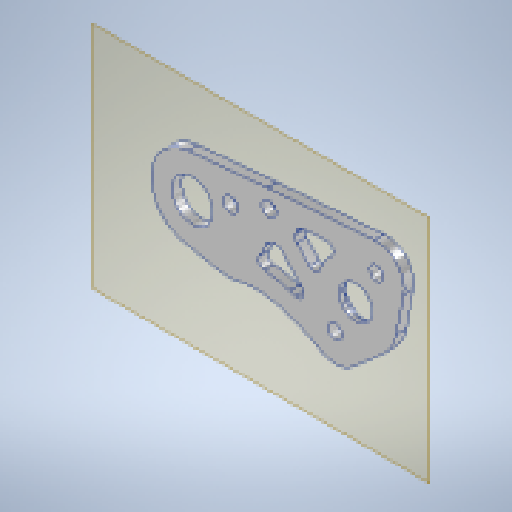
# Autodesk Inventor part: IntakeBearingBlock
Saved by Autodesk Inventor 2023 (Build 270158000, 158)
## iProperties
Created: 2022-11-10
Part Number: IntakeBearingBlock
Material: Aluminum 6061
Document SubType Name: Modeling
Designer: Zac Hah
Density: 2.7 g/cm^3
Appearance: Aluminum - Flat
Author: Zac Hah
Autodesk Inventor part; units mm, degrees
ref_plane "YZ Plane" through (0, 0, 0) normal (1, 0, 0) x (0, 1, 0)
ref_plane "XZ Plane" through (0, 0, 0) normal (0, 1, 0) x (-1, 0, 0)
ref_plane "XY Plane" through (0, 0, 0) normal (0, 0, 1) x (1, 0, 0)
ref_plane "Work Plane1" through (0, 0, 0) normal (0, 0, 1) x (1, 0, 0)
sketch "Sketch1" plane through (0, 0, 0) normal (0, 0, 1) x (1, 0, 0)
  line L0 (44.7498, 2.1658) -> (46.9612, 13.9487) projected
  arc A0 (46.9612, 13.9487) -> (42.8396, 22.8948) centre (38.5982, 15.5182) ccw projected
  arc A1 (42.8396, 22.8948) -> (22.886, 31.7216) centre (-8.8802, -67.0551) ccw projected
  arc A2 (22.886, 31.7216) -> (13.5715, 28.8544) centre (20.2809, 23.6211) ccw projected
  arc A3 (0.8003, 20.1348) -> (13.5715, 28.8544) centre (-6.4566, 44.4761) ccw projected
  line L1 (0.8003, 20.1348) -> (-28.9641, 11.2611) projected
  arc A4 (-28.9641, 11.2611) -> (-47.1072, -13.0801) centre (-21.7072, -13.0801) ccw projected
  line L2 (-47.1072, -13.0801) -> (-47.1072, -25.7801) projected
  arc A5 (-47.1072, -25.7801) -> (-40.7572, -32.1301) centre (-40.7572, -25.7801) ccw projected
  line L3 (-40.7572, -32.1301) -> (-28.0572, -32.1301) projected
  arc A6 (-28.0572, -32.1301) -> (-21.7072, -25.7801) centre (-28.0572, -25.7801) ccw projected
  line L4 (-21.7072, -25.7801) -> (-21.7072, -15.4467) projected
  arc A7 (-19.4393, -12.404) -> (-21.7072, -15.4467) centre (-18.5322, -15.4467) ccw projected
  line L5 (-19.4393, -12.404) -> (-5.7048, -8.3094) projected
  arc A8 (9.7562, -8.6121) -> (-5.7048, -8.3094) centre (1.552, -32.6506) ccw projected
  arc A9 (9.7562, -8.6121) -> (9.8996, -8.6596) centre (12.5046, -0.5592) ccw projected
  arc A10 (21.6959, -13.8779) -> (9.8996, -8.6596) centre (-8.8802, -67.0551) ccw projected
  arc A11 (21.6959, -13.8779) -> (31.501, -12.9394) centre (25.9373, -6.5014) ccw projected
  line L6 (31.501, -12.9394) -> (40.5717, -5.1006) projected
  arc A12 (40.5717, -5.1006) -> (44.7498, 2.1658) centre (32.2678, 4.5084) ccw projected
  arc A13 (29.1025, -0.9965) -> (35.433, 10.0133) centre (32.2678, 4.5084) ccw projected
  arc A14 (29.1025, -0.9965) -> (14.4487, 5.4859) centre (-8.8802, -67.0551) ccw construction
  arc A15 (18.3368, 17.5761) -> (14.4487, 5.4859) centre (16.3928, 11.531) ccw projected
  arc A16 (35.433, 10.0133) -> (18.3368, 17.5761) centre (-8.8802, -67.0551) ccw construction
  arc A17 (24.8611, -8.373) -> (11.8436, -2.6145) centre (-8.8802, -67.0551) ccw construction
  arc A18 (13.1656, 1.4961) -> (11.8436, -2.6145) centre (12.5046, -0.5592) ccw projected
  arc A19 (27.0135, -4.6297) -> (13.1656, 1.4961) centre (-8.8802, -67.0551) ccw construction
  arc A20 (24.8611, -8.373) -> (27.0135, -4.6297) centre (25.9373, -6.5014) ccw projected
  arc A21 (37.5221, 13.6465) -> (39.6744, 17.3899) centre (38.5982, 15.5182) ccw projected
  arc A22 (37.5221, 13.6465) -> (19.6199, 21.5658) centre (-8.8802, -67.0551) ccw construction
  arc A23 (20.9419, 25.6765) -> (19.6199, 21.5658) centre (20.2809, 23.6211) ccw projected
  arc A24 (39.6744, 17.3899) -> (20.9419, 25.6765) centre (-8.8802, -67.0551) ccw construction
  circle A25 centre (-28.0572, -25.7801) radius 2.159 projected
  circle A26 centre (-40.7572, -25.7801) radius 2.159 projected
  circle A27 centre (-40.7572, -13.0801) radius 2.159 projected
  circle A28 centre (-28.0572, -13.0801) radius 2.159 projected
  circle A29 centre (32.2678, 4.5084) radius 6.35
  circle A30 centre (25.9373, -6.5014) radius 2.159
  circle A31 centre (38.5982, 15.5182) radius 2.159
  circle A32 centre (25.9373, -6.5014) radius 8.509
  circle A33 centre (32.2678, 4.5084) radius 12.7
  circle A34 centre (38.5982, 15.5182) radius 8.509
  line L7 (23.9638, 14.1175) -> (33.0346, 21.9563)
  line L8 (19.7857, 6.851) -> (17.5743, -4.9318)
  circle A35 centre (-6.3214, 11.2784) radius 12.7 construction
  circle A36 centre (-6.3214, 11.2784) radius 2.286
  circle A37 centre (5.4641, 16.0103) radius 2.286
  line L9 (5.4641, 16.0103) -> (-18.107, 6.5465) construction
  circle A38 centre (-18.107, 6.5465) radius 6.35
  circle A39 centre (5.4641, 16.0103) radius 5.461
  circle A40 centre (-18.107, 6.5465) radius 17.78 construction
  line L10 (5.0426, 21.455) -> (37.9415, 24.0018)
  line L11 (-19.2837, 19.1919) -> (4.9581, 21.4478)
  line L12 (-28.3337, -10.6773) -> (24.7622, 10.6406) construction
  line L13 (24.7622, 10.6406) -> (15.6909, 33.2342) construction
  line L14 (15.6909, 33.2342) -> (-37.405, 11.9162) construction
  line L15 (-37.405, 11.9162) -> (-28.3337, -10.6773) construction
  line L16 (-28.3337, -10.6773) -> (15.6909, 33.2342) construction
  line L17 (24.7622, 10.6406) -> (-37.405, 11.9162) construction
  circle A41 centre (-18.107, 6.5465) radius 12.7
  line L18 (24.2748, -14.8464) -> (-20.5883, -5.9087)
  point P0 (0, 0)
  point P1 (35.433, 10.0133)
  point P2 (29.1025, -0.9965)
  point P3 (42.8396, 22.8948)
  point P4 (21.6959, -13.8779)
  point P5 (24.8611, -8.373)
  point P6 (21.6959, -13.8779)
  point P7 (-13.0272, -10.4924)
  point P8 (-35.8245, 8.0353)
  point P9 (5.5648, 21.4955)
  point P10 (3.3547, 21.0475)
  point P11 (-4.8892, 18.4386)
  point P12 (4.0842, 21.3665)
  point P13 (42.8396, 22.8948)
  point P14 (30.227, 17.0434)
  point P15 (44.1277, 9.0507)
  point P16 (34.3085, -8.0265)
  point P17 (20.4079, -0.0339)
  point P18 (-6.8397, -8.6477)
  point P19 (31.5086, 10.8129)
  point P20 (38.0983, 7.0239)
  point P21 (40.3716, 14.2868)
  point P22 (36.6419, 16.4314)
  point P23 (27.8937, -7.4145)
  point P24 (33.0269, -1.796)
  point P25 (26.4373, 1.9929)
  point P26 (24.1639, -5.27)
  dimension "d5" = 25.4
  dimension "d6" = 4.572
  dimension "d7" = 4.572
  dimension "d8" = 12.7
  dimension "d9" = 3.175
  dimension "d10" = 11.43
  dimension "d23" = 25.4
  constraints: 24 end point, 15 point on circle, 13 tangent, 11 centre point, 10 coincident, 3 midpoint, 2 parallel, 2 perpendicular, 1 concentric, 1 point on line, 6 other
  measures "d5" diameter of A35
  measures "d6" diameter of A36
  measures "d7" diameter of A37
  measures "d8" diameter of A38
  measures "d9" radial gap between concentric circles of A37 A39
  measures "d10" radial gap between concentric circles of A38 A40
  measures "d23" diameter of A41
extrude "Extrusion1" add sketch "Sketch1" along normal blind 3 contours A33 A34 L0 | A12 A33 A32 A13 A34 | A34 A33 A21 A31 A0 | L6 A32 A33 | A34 A13 A29 A33 A31 A21 | A11 A32 A33 A30 A20 | A33 A20 A30 A32 A29 A13 | A34 L7 A33 L8 A32 A10 A9 A8 L5 L18 A41 A36 L1 A3 A39 L10 | A29 A32 A33 A34 | A34 A33 L7 | L8 A33 A32 | A41 A4 L1 A36 | L11 A39 A3 | A3 L1 A41 L11 | A39 | A41 L1 A4
sketch "Sketch2" plane through (0, 0, 3) normal (0, 0, 1) x (1, 0, 0)
  arc A0 (38.0983, 7.0239) -> (38.0983, 7.0239) centre (32.2678, 4.5084) ccw projected
  circle A1 centre (32.2678, 4.5084) radius 5.08
  circle A2 centre (32.2678, 4.5084) radius 6.35
  point P0 (0, 0)
  dimension "d2" = 1.27
  constraints: 2 centre point, 2 coincident
  measures "d2" radial gap between concentric circles of A0 A1
extrude "Extrusion2" add sketch "Sketch2" against normal blind 1.3716
sketch "Sketch3" plane through (0, 0, 3) normal (0, 0, 1) x (1, 0, 0)
  arc A0 (40.5717, -5.1006) -> (44.7498, 2.1658) centre (32.2678, 4.5084) ccw projected
  line L0 (44.7498, 2.1658) -> (46.9612, 13.9487) projected
  arc A1 (46.9612, 13.9487) -> (37.9415, 24.0018) centre (38.5982, 15.5182) ccw projected
  line L1 (-6.8397, -8.6477) -> (-5.7048, -8.3094) projected
  arc A2 (9.7562, -8.6121) -> (-5.7048, -8.3094) centre (1.552, -32.6506) ccw projected
  arc A3 (9.7562, -8.6121) -> (9.8996, -8.6596) centre (12.5046, -0.5592) ccw projected
  arc A4 (21.6959, -13.8779) -> (9.8996, -8.6596) centre (-8.8802, -67.0551) ccw projected
  arc A5 (21.6959, -13.8779) -> (31.501, -12.9394) centre (25.9373, -6.5014) ccw projected
  line L2 (31.501, -12.9394) -> (40.5717, -5.1006) projected
  circle A6 centre (25.9373, -6.5014) radius 2.159 projected
  circle A7 centre (38.5982, 15.5182) radius 2.159 projected
  line L3 (-37.7734, 20.5283) -> (5.443, 15.117)
  line L4 (5.443, 15.117) -> (38.4316, 17.6708)
  arc A8 (40.7202, 15.12) -> (38.4316, 17.6708) centre (38.5982, 15.5182) ccw
  line L5 (40.7202, 15.12) -> (38.5088, 3.3371)
  arc A9 (36.4198, -0.2961) -> (38.5088, 3.3371) centre (32.2678, 4.5084) ccw
  line L6 (36.4198, -0.2961) -> (27.349, -8.1349)
  arc A10 (24.8611, -8.373) -> (27.349, -8.1349) centre (25.9373, -6.5014) ccw
  arc A11 (24.8611, -8.373) -> (11.8436, -2.6145) centre (-8.8802, -67.0551) ccw
  arc A12 (11.8073, -2.6025) -> (11.8436, -2.6145) centre (12.5046, -0.5592) ccw
  arc A13 (11.8073, -2.6025) -> (-7.5191, -2.224) centre (1.552, -32.6506) ccw
  line L7 (-7.5191, -2.224) -> (-35.2068, -10.4786)
  arc A14 (-37.7734, 20.5283) -> (-35.2068, -10.4786) centre (-18.107, 6.5465) ccw
  circle A15 centre (32.2678, 4.5084) radius 11.43
  circle A16 centre (25.9373, -6.5014) radius 8.509
  circle A17 centre (38.5982, 15.5182) radius 8.509
  circle A18 centre (5.4641, 16.0103) radius 8.636
  circle A19 centre (-4.0855, 7.638) radius 8.636
  circle A20 centre (-13.635, -0.7343) radius 12.7
  line L8 (25.9373, -6.5014) -> (5.4641, 16.0103) construction
  line L9 (28.2862, -4.3652) -> (7.813, 18.1465)
  line L10 (3.1152, 13.8741) -> (23.5884, -8.6375)
  arc A21 (23.5884, -8.6375) -> (28.2862, -4.3652) centre (25.9373, -6.5014) ccw
  arc A22 (7.813, 18.1465) -> (3.1152, 13.8741) centre (5.4641, 16.0103) ccw
  line L11 (37.9415, 24.0018) -> (5.0426, 21.455) projected
  arc A23 (5.0426, 21.455) -> (4.9581, 21.4478) centre (5.4641, 16.0103) ccw projected
  line L12 (4.9581, 21.4478) -> (-19.2837, 19.1919) projected
  arc A24 (-19.2837, 19.1919) -> (-20.5883, -5.9087) centre (-18.107, 6.5465) ccw projected
  line L13 (-20.5883, -5.9087) -> (-6.8397, -8.6477) projected
  point P0 (0, 0)
  point P1 (15.7007, 4.7545)
  point P2 (13.2165, 12.205)
  point P3 (20.8597, 3.8008)
  point P4 (30.0919, 15.7294)
  point P5 (30.2256, 17.0355)
  point P6 (14.0972, 15.787)
  point P7 (17.608, -4.7619)
  point P8 (18.2769, -2.7972)
  point P9 (8.5188, 7.9326)
  point P10 (4.5479, 7.4231)
  point P11 (-0.9393, -0.4045)
  point P12 (-0.9378, -0.9984)
  dimension "d13" = 6.35
  dimension "d14" = 6.35
  dimension "d18" = 6.35
  constraints: 18 end point, 18 point on circle, 15 centre point, 4 tangent, 1 midpoint, 1 parallel, 8 other
  measures "d13" radial gap between concentric circles of A6 A16
  measures "d14" radial gap between concentric circles of A7 A17
  measures "d18" diameter of A22
extrude "Extrusion3" cut sketch "Sketch3" against normal blind 3 contours A11 A12 A13 A20 A19 A18 L10 A16 | A17 A15 L9 A18 L4
fillet "Fillet1" radius 2 11 edges at (30.2256, 17.0355, 1.5) (30.0919, 15.7294, 1.5) (14.0972, 15.787, 1.5) (13.2165, 12.205, 1.5) (20.8597, 3.8008, 1.5) (18.2769, -2.7972, 1.5) (17.608, -4.7619, 1.5) (8.5188, 7.9326, 1.5) (4.5479, 7.4231, 1.5) (-0.9393, -0.4045, 1.5) (-0.9378, -0.9984, 1.5)
fillet "Fillet2" radius 12.7 1 edges at (-6.8397, -8.6477, 1.5)
body "Solid1"
